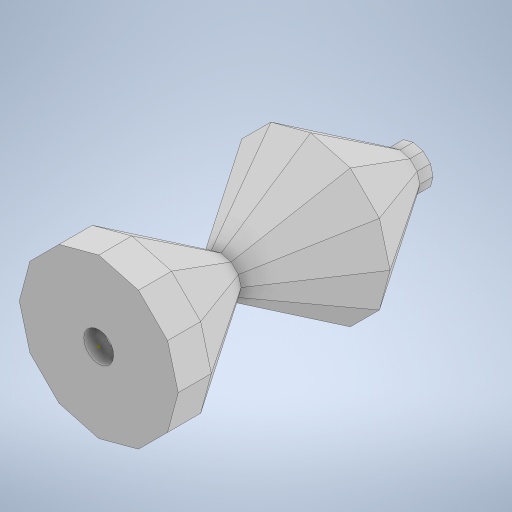
# Autodesk Inventor part: Test27
Saved by Autodesk Inventor 2023 (Build 270158000, 158)
## iProperties
Created: 2024-07-02
Part Number: Test27
Material: 일반
Document SubType Name: Modeling
Designer: ojs08
Density: 1 g/cm^3
Appearance: 기본값
Author: ojs08
Autodesk Inventor part; units mm, degrees
ref_plane "YZ Plane" through (0, 0, 0) normal (1, 0, 0) x (0, 1, 0)
ref_plane "XZ Plane" through (0, 0, 0) normal (0, 1, 0) x (-1, 0, 0)
sketch "스케치1" plane through (0, 0, 0) normal (0, 0, 1) x (1, 0, 0)
  line L0 (10.392305, 6) -> (12, 0)
  line L1 (12, 0) -> (10.392305, -6)
  line L2 (10.392305, -6) -> (6, -10.392305)
  line L3 (6, -10.392305) -> (0, -12)
  line L4 (0, -12) -> (-6, -10.392305)
  line L5 (-6, -10.392305) -> (-10.392305, -6)
  line L6 (-10.392305, -6) -> (-12, 0)
  line L7 (-12, 0) -> (-10.392305, 6)
  line L8 (-10.392305, 6) -> (-6, 10.392305)
  line L9 (-6, 10.392305) -> (0, 12)
  line L10 (0, 12) -> (6, 10.392305)
  line L11 (6, 10.392305) -> (10.392305, 6)
  line L12 (-16.8, 0) -> (16.8, 0)
  point P0 (0, 0)
  point P1 (0, 0)
  dimension "d0" = 24
  constraints: 24 end point, 1 coincident, 1 point on line, 25 other
  measures "d0" distance of L0.end L6.end
ref_plane "작업 평면1" through (0, 0, 13.5) normal (0, 0, 1) x (1, 0, 0)
sketch "스케치2" plane through (0, 0, 13.5) normal (0, 0, 1) x (1, 0, 0)
  line L0 (2.598076, 1.5) -> (3, 0)
  line L1 (3, 0) -> (2.598076, -1.5)
  line L2 (2.598076, -1.5) -> (1.5, -2.598076)
  line L3 (1.5, -2.598076) -> (0, -3)
  line L4 (0, -3) -> (-1.5, -2.598076)
  line L5 (-1.5, -2.598076) -> (-2.598076, -1.5)
  line L6 (-2.598076, -1.5) -> (-3, 0)
  line L7 (-3, 0) -> (-2.598076, 1.5)
  line L8 (-2.598076, 1.5) -> (-1.5, 2.598076)
  line L9 (-1.5, 2.598076) -> (0, 3)
  line L10 (0, 3) -> (1.5, 2.598076)
  line L11 (1.5, 2.598076) -> (2.598076, 1.5)
  line L12 (-4.2, 0) -> (4.2, 0)
  point P0 (0, 0)
  point P1 (0, 0)
  dimension "d2" = 6
  constraints: 24 end point, 1 coincident, 1 point on line, 25 other
  measures "d2" distance of L0.end L6.end
loft "로프트1" add profiles "스케치1", "스케치2"
mirror "미러1" about plane through (0, 0, 13.5) normal (0, 0, 1) of "로프트1"
mirror "미러2" about plane through (0, 0, 0) normal (0, 0, -1) of "로프트1"
sketch "스케치7" plane through (12, 0, 27) normal (0, 0, 1) x (0.9659258, 0.258819, 0)
  line L0 (0, 6.211657) -> (0, 0)
  line L1 (-3.105829, 11.59111) -> (0, 6.211657)
  line L2 (-8.485281, 14.696938) -> (-3.105829, 11.59111)
  line L3 (-14.696938, 14.696938) -> (-8.485281, 14.696938)
  line L4 (-20.076391, 11.59111) -> (-14.696938, 14.696938)
  line L5 (-23.18222, 6.211657) -> (-20.076391, 11.59111)
  line L6 (-23.18222, 0) -> (-23.18222, 6.211657)
  line L7 (-20.076391, -5.379453) -> (-23.18222, 0)
  line L8 (-14.696938, -8.485281) -> (-20.076391, -5.379453)
  line L9 (-8.485281, -8.485281) -> (-14.696938, -8.485281)
  line L10 (-3.105829, -5.379453) -> (-8.485281, -8.485281)
  line L11 (0, 0) -> (-3.105829, -5.379453)
  point P0 (-11.59111, 3.105829)
extrude "돌출5" add sketch "스케치7" along normal blind 2.5
shell "쉘2" thickness 0.5 removed faces 0 ; own thickness 2 on faces at (-7.171633, -7.171633, -2.25) (-2.625, -9.796633, -2.25) (-9.796633, -2.625, -2.25) (-9.796633, 2.625, -2.25) (-7.171633, 7.171633, -2.25) (7.171633, 7.171633, -2.25) (2.625, 9.796633, -2.25) (-2.625, 9.796633, -2.25) (9.796633, 2.625, -2.25) (9.796633, -2.625, -2.25) (7.171633, -7.171633, -2.25) (2.625, -9.796633, -2.25) (-9.796633, 2.625, 24.75) (-7.171633, 7.171633, 24.75) (-2.625, 9.796633, 24.75) (2.625, 9.796633, 24.75) (7.171633, 7.171633, 24.75) (9.796633, 2.625, 24.75) (9.796633, -2.625, 24.75) (7.171633, -7.171633, 24.75) (-2.625, -9.796633, 24.75) (2.625, -9.796633, 24.75) (-7.171633, -7.171633, 24.75) (-9.796633, -2.625, 24.75)
sketch "스케치8" plane through (12, 0, 29.5) normal (0, 0, 1) x (0.9659258, 0.258819, 0)
  line L0 (-3.105829, 11.59111) -> (-8.485281, 14.696938)
  line L1 (-8.485281, 14.696938) -> (-14.696938, 14.696938)
  line L2 (-14.696938, 14.696938) -> (-20.076391, 11.59111)
  line L3 (-20.076391, 11.59111) -> (-23.18222, 6.211657)
  line L4 (-23.18222, 6.211657) -> (-23.18222, 0)
  line L5 (-23.18222, 0) -> (-20.076391, -5.379453)
  line L6 (-20.076391, -5.379453) -> (-14.696938, -8.485281)
  line L7 (-14.696938, -8.485281) -> (-8.485281, -8.485281)
  line L8 (-8.485281, -8.485281) -> (-3.105829, -5.379453)
  line L9 (-3.105829, -5.379453) -> (0, 0)
  line L10 (0, 0) -> (0, 6.211657)
  line L11 (0, 6.211657) -> (-3.105829, 11.59111)
  point P0 (-11.59111, 3.105829)
extrude "돌출6" add sketch "스케치8" along normal blind 2.5
sketch "스케치9" plane through (12, 0, 32) normal (0, 0, 1) x (0.9659258, 0.258819, 0)
  circle A0 centre (-11.59111, 3.105829) radius 2.25
  point P0 (-11.59111, 3.105829)
  dimension "d24" = 4.5
  constraints: 1 centre point, 1 coincident
  measures "d24" diameter of A0
sketch "스케치10" plane through (12, 0, 32) normal (0, 0, 1) x (0.9659258, 0.258819, 0)
  point P0 (-11.59111, 3.105829)
extrude "돌출7" cut sketch "스케치9" against normal blind 3
sketch "스케치11" plane through (3, 0, -13.5) normal (0, 0, -1) x (-0.9659258, -0.258819, 0)
  line L0 (0, 1.552914) -> (0, 0)
  line L1 (0, 0) -> (0.776457, -1.344863)
  line L2 (0.776457, -1.344863) -> (2.12132, -2.12132)
  line L3 (2.12132, -2.12132) -> (3.674235, -2.12132)
  line L4 (3.674235, -2.12132) -> (5.019098, -1.344863)
  line L5 (5.019098, -1.344863) -> (5.795555, 0)
  line L6 (5.795555, 0) -> (5.795555, 1.552914)
  line L7 (5.795555, 1.552914) -> (5.019098, 2.897777)
  line L8 (5.019098, 2.897777) -> (3.674235, 3.674235)
  line L9 (3.674235, 3.674235) -> (2.12132, 3.674235)
  line L10 (2.12132, 3.674235) -> (0.776457, 2.897777)
  line L11 (0.776457, 2.897777) -> (0, 1.552914)
  point P0 (2.897777, 0.776457)
extrude "돌출8" add sketch "스케치11" along normal blind 2
